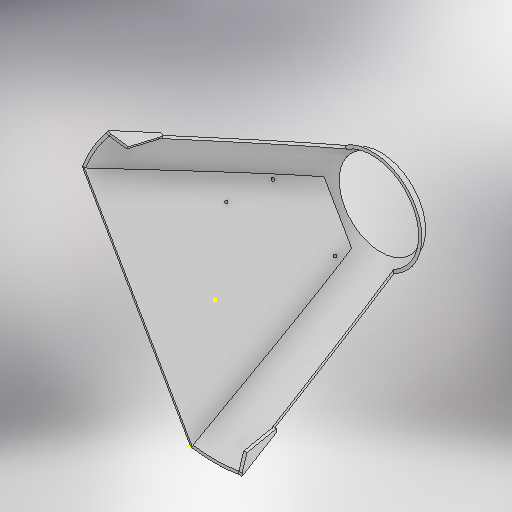
# Autodesk Inventor part: +uno_holder
Saved by Autodesk Inventor 2026.2 (Build 302298000, 298)
## iProperties
Created: 2026-01-13
Part Number: +uno_holder
Material: Generic
Document SubType Name: Modeling
Designer: bjones
Density: 1 g/cm^3
Appearance: Default
Author: bjones
Autodesk Inventor part; units mm, degrees
ref_plane "YZ Plane" through (0, 0, 0) normal (1, 0, 0) x (0, 1, 0)
ref_plane "XZ Plane" through (0, 0, 0) normal (0, 1, 0) x (-1, 0, 0)
ref_plane "XY Plane" through (0, 0, 0) normal (0, 0, 1) x (1, 0, 0)
ref_plane "Work Plane1" through (0, 0, 0) normal (0, 0, 1) x (1, 0, 0)
sketch "Sketch1" plane through (0, 0, 0) normal (0, 0, 1) x (1, 0, 0)
  arc A0 (94.279275, 34.299578) -> (77.023762, 64.283612) centre (0, 0) ccw
  circle A1 centre (0, 0) radius 102.610686
  point P0 (0, 0)
  constraints: 1 centre point
ref_plane "Work Plane2" through (-14.496752, 26.793437, -120.65) normal (0, 0, -1) x (-1, 0, 0)
sketch "Sketch2" plane through (-14.496752, 26.793437, -120.65) normal (0, 0, -1) x (-1, 0, 0)
  circle A0 centre (-14.496752, -26.793437) radius 32.547518
  point P0 (-14.496752, -26.793437)
  constraints: 1 centre point
loft "Loft1" add profiles "Sketch1", "Sketch2"
shell "Shell1" thickness 2.159 removed faces 0
sketch "Sketch3" plane through (0, 0, 0) normal (0, 0, 1) x (1, 0, 0)
  circle A0 centre (0, 0) radius 100.451686
  point P0 (0, 0)
  constraints: 1 centre point
sketch "Sketch4" plane through (-14.496752, 26.793437, -120.65) normal (0, 0, -1) x (-1, 0, 0)
  circle A0 centre (-14.496752, -26.793437) radius 30.261518
  point P0 (-14.496752, -26.793437)
  constraints: 1 centre point
loft "Loft2" cut profiles "Sketch3", "Sketch4"
sketch "Sketch5" plane through (0, 0, 0) normal (0, 0, 1) x (1, 0, 0)
  arc A0 (-17.006258, -88.621363) -> (16.758707, -88.668509) centre (0, 0) ccw
  line L0 (17.163344, -99.043842) -> (16.944697, -88.206273)
  line L1 (-17.190957, -88.158609) -> (-17.439868, -98.995525)
  line L2 (-15.779285, -26.698255) -> (-17.190957, -88.158609)
  line L3 (16.944697, -88.206273) -> (15.704665, -26.742216)
  line L4 (-84.861222, 29.428598) -> (-31.011771, -0.229531)
  line L5 (-94.356155, 34.658029) -> (-84.861222, 29.428598)
  line L6 (-15.231724, 27.014389) -> (-67.752117, 58.96711)
  line L7 (-67.752117, 58.96711) -> (-77.012706, 64.601131)
  circle A1 centre (0, 0) radius 100.451686
  arc A2 (-68.245223, 59.038532) -> (-85.168535, 29.820789) centre (0, 0) ccw
  arc A3 (-30.224841, -1.489446) -> (-16.473272, -25.384853) centre (0, 0) ccw
  arc A4 (13.822523, 26.920203) -> (-13.747291, 26.958699) centre (0, 0) ccw
  circle A5 centre (0, 0) radius 30.261518
  circle A6 centre (0, 0) radius 102.610686
  line L8 (17.163344, -99.043842) -> (17.163344, -101.165076)
  line L9 (-17.439868, -98.995525) -> (-17.439868, -101.117773)
  line L10 (-77.012706, 64.601131) -> (-78.819087, 65.70011)
  line L11 (-94.356155, 34.658029) -> (-96.208248, 35.678088)
  line L12 (15.704665, -26.742216) -> (15.704665, -25.867411)
  line L13 (-15.231724, 27.014389) -> (-14.493251, 26.565111)
  line L14 (-31.251349, -0.097581) -> (-30.25461, -0.646545)
  line L15 (-15.779285, -26.698255) -> (-15.779285, -25.82196)
  point P0 (-94.295657, 34.624709)
  point P1 (-17.438282, -98.926476)
  point P2 (17.161951, -98.974788)
  point P3 (-76.9537, 64.565233)
  constraints: 16 end point, 4 collinear, 4 point on circle, 4 vertical, 1 point on line, 5 other
extrude "Extrusion1" cut sketch "Sketch5" against normal blind 114.3 contours L0 A1 L7 L10 A6 L8 | L0 L3 L12 A5 A4 L13 L6 L7 A1 | A1 L5 L4 L14 A5 A3 L15 L2 L1 | L1 L9 A6 L11 L5 A1
ref_plane "Work Plane3" through (-17.439868, -101.117773, 0) normal (0.8276743, 0.4763183, 0.2967762) x (0.0114489, 0.5143752, -0.8574888)
sketch "Sketch6" plane through (-17.439868, -101.117773, 0) normal (0.8276743, 0.4763183, 0.2967762) x (0.0114489, 0.5143752, -0.8574888)
  ellipse E0 centre (150.223115, 14.285442) end of major axis (166.170528, 46.822484) minor radius 10.753703 (133.636756, -17.838738) -> (165.452784, 47.074577) ccw
  line L0 (134.59672, 1.769523) -> (133.296202, 0)
  spline S0 degree 2 poles (151.144629, 36.415626) (131.405277, 63.131418) (69.462591, 141.748059) knots 0 0 0 1 1 1 weights 1 1.15005095 1
  spline S1 degree 2 poles (4.178817, 0.000291) (100.619816, -0.752262) (133.296202, 0) knots 0 0 0 1 1 1 weights 1 1.1442006 1
  spline S2 degree 2 poles (0, 0) (2.111396, -0.00009) (4.178817, 0.000291) knots 0 0 0 1 1 1 weights 1 1.00005458 1
  line L1 (0, 0) -> (69.462591, 141.748059)
  line L2 (133.296202, 0) -> (151.144629, 36.415626)
  point P0 (52.212145, 62.323656)
  constraints: 4 end point, 4 other
extrude "Extrusion2" add sketch "Sketch6" along normal blind 2.286
sketch "Sketch8" plane through (17.163344, -101.165076, 0) normal (0, 0, 1) x (1, 0, 0)
  point P0 (-17.163344, 101.165076)
sketch "Sketch9" plane through (17.163344, -99.043842, 0) normal (0.9997965, 0.0201708, 0) x (0, 0, -1)
  spline S0 degree 2 poles (0, 0.069067) (87.521453, 51.576258) (114.3, 68.987261) knots 0 0 0 1 1 1 weights 1 1.1647756 1
  spline S1 degree 2 poles (114.3, 66.459541) (86.758721, 48.850205) (3.600262, 0) knots 0 0 0 1 1 1 weights 1 1.1442006 1
  spline S2 degree 2 poles (3.600262, 0) (1.819204, -1.049487) (0, -2.120803) knots 0 0 0 1 1 1 weights 1 1.00005453 1
  line L0 (0, -2.120803) -> (0, 0)
  line L1 (25.4, 12.827487) -> (25.4, 15.047384)
  line L2 (0, 0.069067) -> (0, -2.120803)
  point P0 (0, 99.369889)
  point P1 (25.4, 13.937436)
  point P2 (0, -1.060401)
  point P3 (0, 0)
  dimension "d19" = 25.4
  constraints: 4 end point, 2 midpoint, 1 collinear, 1 parallel, 1 vertical, 5 other
  measures "d19" horizontal distance of point (25.4, 13.937) point (0, -1.06)
extrude "Extrusion4" add sketch "Sketch9" along normal blind 0.381
sketch "Sketch10" plane through (17.544267, -99.036156, 0) normal (0.9997965, 0.0201708, 0) x (0, 0, -1)
  spline S0 degree 2 poles (3.600262, 0) (15.252195, 6.844755) (25.4, 12.827487) knots 0 0 0 1 1 1 weights 1 1.01797604 1.03147029
  line L0 (25.4, 12.827487) -> (25.4, 15.047384)
  line L1 (0, 0.069067) -> (0, -2.120803)
  spline S1 degree 2 poles (0, -2.120803) (1.819204, -1.049487) (3.600262, 0) knots 0 0 0 1 1 1 weights 1 1.00005453 1
  line L2 (0, 0.069067) -> (3.800675, 10.719427)
  line L3 (3.800675, 10.719427) -> (25.4, 15.047384)
  point P0 (0, 99.369889)
  constraints: 4 end point, 3 other
extrude "Extrusion5" add sketch "Sketch10" along normal blind 2.286
sketch "Sketch11" plane through (-17.439868, -101.117773, 0) normal (-0.8276743, -0.4763183, -0.2967762) x (-0.0114489, -0.5143752, 0.8574888)
  circle A0 centre (-124.378724, 4.590572) radius 1.5875
  circle A1 centre (-131.874338, 57.260258) radius 1.5875
  circle A2 centre (-106.576028, 69.260071) radius 1.5875
  circle A3 centre (-124.378724, 4.590572) radius 2.965293
  circle A4 centre (-131.874338, 57.260258) radius 3.172298
  circle A5 centre (-106.576028, 69.260071) radius 2.694207
  circle A6 centre (-124.378724, 4.590572) radius 1.016
  circle A7 centre (-131.874338, 57.260258) radius 1.016
  circle A8 centre (-106.576028, 69.260071) radius 1.016
  point P0 (-52.212145, 62.323656)
  dimension "d24" = 2.032
  dimension "d25" = 2.032
  dimension "d26" = 2.032
  constraints: 9 centre point, 6 coincident, 6 other
  measures "d24" diameter of A6
  measures "d25" diameter of A7
  measures "d26" diameter of A8
extrude "Extrusion6" add sketch "Sketch11" along normal blind 3.048 contours A0 | A1 | A2 | A3 | A4 | A5
sketch "Sketch12" plane through (0, 0, -114.3) normal (0, 0, 1) x (1, 0, 0)
  arc A0 (-36.141943, 2.595963) -> (-15.913773, -32.553508) centre (0, 0) ccw
  line L0 (-18.122715, -28.71514) -> (-33.933, -1.242405)
  line L1 (-36.141943, 2.595963) -> (-33.933, -1.242405)
  line L2 (-18.122715, -28.71514) -> (-15.913773, -32.553508)
  point P0 (0, 0)
extrude "Extrusion7" add sketch "Sketch12" along normal blind 2.286
sketch "Sketch14" plane through (-17.439868, -101.117773, 0) normal (-0.8276743, -0.4763183, -0.2967762) x (-0.0114489, -0.5143752, 0.8574888)
  circle A0 centre (-131.874338, 57.260258) radius 1.016
  line L0 (-131.874338, 57.260258) -> (-138.666491, 53.806121)
  line L1 (-132.564429, 60.356586) -> (-69.445188, 141.686996)
  line L2 (-138.666491, 53.806121) -> (-139.127042, 54.711741)
  line L3 (-139.127042, 54.711741) -> (-135.02107, 56.799826)
  line L4 (-138.666491, 53.806121) -> (-138.205939, 52.900501)
  line L5 (-138.205939, 52.900501) -> (-134.107025, 54.984996)
  arc A1 (-135.02107, 56.799826) -> (-134.107025, 54.984996) centre (-131.654503, 57.357812) ccw
  circle A2 centre (-106.576028, 69.260071) radius 1.016
  circle A3 centre (-124.378724, 4.590572) radius 1.016
  line L6 (-105.560028, 69.728072) -> (-112.352181, 66.273936)
  line L7 (-112.352181, 66.273936) -> (-112.812732, 67.179556)
  line L8 (-112.812732, 67.179556) -> (-108.70676, 69.267641)
  line L9 (-111.891629, 65.368315) -> (-107.792715, 67.45281)
  line L10 (-112.352181, 66.273936) -> (-111.891629, 65.368315)
  arc A4 (-108.70676, 69.267641) -> (-107.792715, 67.45281) centre (-105.340193, 69.825626) ccw
  line L11 (-123.375776, 4.752904) -> (-130.167929, 1.298767)
  line L12 (-130.167929, 1.298767) -> (-130.628481, 2.204388)
  line L13 (-130.628481, 2.204388) -> (-126.522508, 4.292473)
  line L14 (-129.707377, 0.393147) -> (-125.608463, 2.477642)
  line L15 (-130.167929, 1.298767) -> (-129.707377, 0.393147)
  arc A5 (-126.522508, 4.292473) -> (-125.608463, 2.477642) centre (-123.155941, 4.850458) ccw
  point P0 (-52.212145, 62.323656)
  constraints: 30 end point, 6 point on circle, 3 centre point, 3 parallel, 3 perpendicular, 3 symmetric about line
extrude "Extrusion8" add sketch "Sketch14" along normal up to surface (3.048 mm away) contours A1 L5 L4 L0 | L0 L2 L3 A1 | A4 L9 L10 L6 | L6 L7 L8 A4 | A5 L14 L15 L11 | L11 L12 L13 A5
chamfer "Chamfer1" distance 3.048 angle 45 3 edges at (-55.8621, 2.4828, -69.3916) (-48.5652, 7.1272, -97.1958) (-19.2011, -34.6883, -111.9763)
sketch "Sketch15" plane through (-17.439868, -101.117773, 0) normal (-0.8276743, -0.4763183, -0.2967762) x (-0.0114489, -0.5143752, 0.8574888)
  line L0 (-69.462591, 141.748059) -> (0, 0)
  line L1 (-34.731296, 70.87403) -> (-142.220415, 18.207813)
  line L2 (-133.368997, 0.148522) -> (-151.071833, 36.267104)
  point P0 (-52.212145, 62.323656)
  constraints: 2 end point, 2 midpoint
ref_plane "Work Plane4" through (-56.809081, -32.711223, 0.00537) normal (-0.4988241, 0.8667032, 0.0001256) x (0.2571571, 0.1481431, -0.954947)
mirror "Mirror1" about plane through (-56.809081, -32.711223, 0.00537) normal (-0.4988241, 0.8667032, 0.0001256) of "Extrusion5", "Extrusion4"
sketch "Sketch17" plane through (-17.439868, -101.117773, 0) normal (-0.8276743, -0.4763183, -0.2967762) x (-0.0114489, -0.5143752, 0.8574888)
  circle A0 centre (-106.576028, 69.260071) radius 1.016
  circle A1 centre (-131.874338, 57.260258) radius 1.016
  circle A2 centre (-124.378724, 4.590572) radius 1.016
  point P0 (-52.212145, 62.323656)
extrude "Extrusion9" cut sketch "Sketch17" against normal blind 2.54
body "Solid1"
